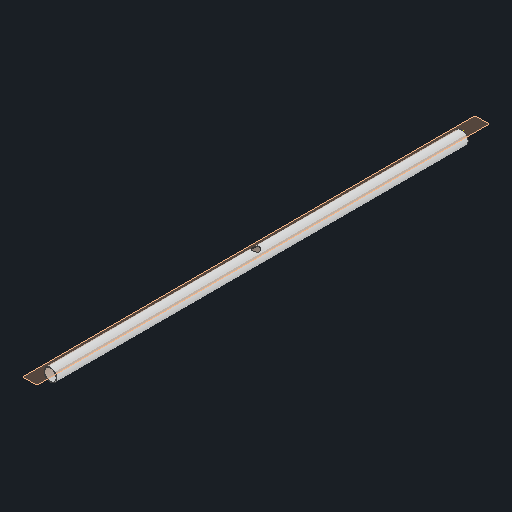
# Autodesk Inventor part: Tubo para aspersores
Saved by Autodesk Inventor 2024 (Build 280153000, 153)
## iProperties
Created: 2024-11-05
Part Number: Tubo para aspersores
Material: Genérico
Document SubType Name: Modeling
Designer: nesto
Density: 1 g/cm^3
Appearance: Valor por defecto
Author: nesto
Autodesk Inventor part; units mm, degrees
ref_plane "YZ Plane" through (0, 0, 0) normal (1, 0, 0) x (0, 1, 0)
ref_plane "XY Plane" through (0, 0, 0) normal (0, 0, 1) x (1, 0, 0)
sketch "Boceto1" plane through (0, 0, 0) normal (0, 0, 1) x (1, 0, 0)
  circle A0 centre (0, 0) radius 95
  circle A1 centre (0, 0) radius 85.31
  dimension "d0" = 190
  dimension "d1" = 170.62
  constraints: 2 centre point, 2 coincident
  measures "d0" diameter of A0
  measures "d1" diameter of A1
extrude "Extrusión1" add sketch "Boceto1" along normal blind 6000
ref_plane "Plano de trabajo4" through (0, 69.75, 0) normal (0, 1, 0) x (-1, 0, 0)
sketch "Boceto5" plane through (0, 69.75, 0) normal (0, 1, 0) x (-1, 0, 0)
  point P0 (0, 0)
sketch "Boceto6" plane through (0, 69.75, 0) normal (0, 1, 0) x (-1, 0, 0)
  line L0 (0, 0) -> (0, 3000) construction
  circle A0 centre (0, 3000) radius 52.5
  dimension "d18" = 105
  constraints: 2 end point, 1 centre point, 1 coincident, 1 vertical
  measures "d18" diameter of A0
extrude "Extrusión5" cut sketch "Boceto6" along normal mid plane 60
